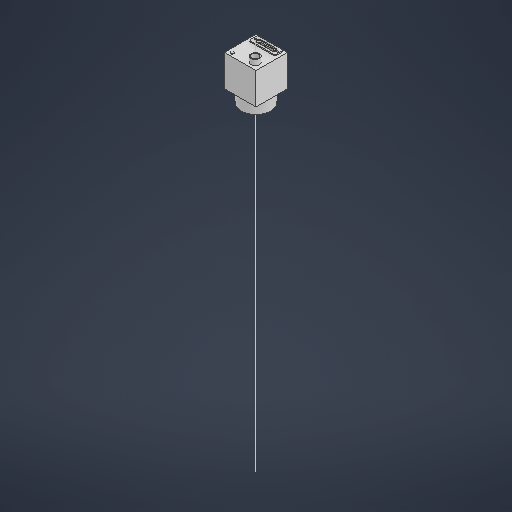
# Autodesk Inventor part: OpticalCamera
Saved by Autodesk Inventor 2026.2 (Build 302298000, 298)
## iProperties
Created: 2026-02-27
Part Number: OpticalCamera
Material: Generic
Document SubType Name: Modeling
Designer: mumin
Density: 1 g/cm^3
Appearance: Default
Author: mumin
Autodesk Inventor part; units mm, degrees
ref_plane "YZ Plane" through (0, 0, 0) normal (1, 0, 0) x (0, 1, 0)
ref_plane "XZ Plane" through (0, 0, 0) normal (0, 1, 0) x (-1, 0, 0)
sketch "Sketch1" plane through (0, 0, 0) normal (0, 1, 0) x (-1, 0, 0)
  line L0 (-15, -15) -> (15, -15)
  line L1 (15, -15) -> (15, 15)
  line L2 (15, 15) -> (-15, 15)
  line L3 (-15, 15) -> (-15, -15)
  line L4 (-15, -15) -> (15, 15) construction
  line L5 (15, -15) -> (-15, 15) construction
  point P0 (0, 0)
  dimension "d0" = 30
  dimension "d1" = 30
  constraints: 12 end point, 2 midpoint, 2 parallel, 1 horizontal, 1 perpendicular
  measures "d0" distance of L2.end L1.end
  measures "d1" distance of L1.end L0.end
extrude "Cube" add sketch "Sketch1" along normal blind 30
sketch "Sketch2" plane through (0, 0, 0) normal (0, -1, 0) x (1, 0, 0)
  circle A0 centre (0, 0) radius 14
  circle A1 centre (0, 0) radius 12.5
  dimension "d4" = 28
  dimension "d7" = 1.5
  constraints: 2 centre point, 1 coincident
  measures "d4" diameter of A0
  measures "d7" radial gap between concentric circles of A0 A1
extrude "Lens Mount" add sketch "Sketch2" along normal blind 11.3
sketch "Sketch3" plane through (0, 0, 0) normal (0, -1, 0) x (1, 0, 0)
  line L0 (7.5, -5) -> (-7.5, -5)
  line L1 (-7.5, -5) -> (-7.5, 5)
  line L2 (-7.5, 5) -> (7.5, 5)
  line L3 (7.5, 5) -> (7.5, -5)
  line L4 (7.5, -5) -> (-7.5, 5) construction
  line L5 (-7.5, -5) -> (7.5, 5) construction
  point P0 (0, 0)
  dimension "d8" = 15
  dimension "d9" = 10
  constraints: 12 end point, 2 midpoint, 2 parallel, 1 horizontal, 1 perpendicular
  measures "d8" distance of L1.end L2.end
  measures "d9" distance of L0.end L1.end
extrude "\"Sensor\"" cut sketch "Sketch3" against normal blind 2
sketch "Sketch4" plane through (15, 0, -15) normal (0, 0, -1) x (-1, 0, 0)
  line L0 (15, 0) -> (15, 30.669)
  line L1 (0, 30) -> (30, 30) projected
  point P0 (15, 26.85)
  point P1 (5, 3.15)
  point P2 (25, 3.15)
  dimension "d12" = 23.7
  dimension "d13" = 20
  dimension "d14" = 3.15
  constraints: 2 end point, 1 point on line, 1 symmetric about line
  measures "d12" vertical distance of point (15, 26.85) point (5, 3.15)
  measures "d13" distance of point (25, 3.15) point (5, 3.15)
  measures "d14" distance from line of L1 point (15, 26.85)
hole "Mounting Holes" at (0, 26.85, -15) at (10, 3.15, -15) at (-10, 3.15, -15) direction (0, 0, 1) diameter 3 depth 3 tip angle 118
sketch "Sketch5" plane through (0, 30, 0) normal (0, 1, 0) x (1, 0, 0)
  circle A0 centre (7.7053, -8.4968) radius 4
  circle A1 centre (7.7053, -8.4968) radius 3.2659
  point P0 (0, 0)
  dimension "d22" = 8
  constraints: 2 centre point
  measures "d22" diameter of A0
extrude "Cable Port" add sketch "Sketch5" along normal blind 5
sketch "Sketch6" plane through (0, 30, 0) normal (0, 1, 0) x (1, 0, 0)
  line L0 (7.2728, 8.793) -> (-7.0273, 8.793)
  line L1 (-7.0273, 8.793) -> (-6.3141, 10.6463)
  line L2 (-6.3141, 10.6463) -> (-2.7583, 10.6463)
  line L3 (-2.7583, 10.6463) -> (-2.3847, 9.4043)
  line L4 (-2.3847, 9.4043) -> (-1.5951, 9.4043)
  line L5 (-1.5951, 9.4043) -> (-1.2927, 10.6463)
  line L6 (-1.2927, 10.6463) -> (6.6007, 10.6463)
  line L7 (6.6007, 10.6463) -> (7.2728, 8.793)
  point P0 (0, 0)
  constraints: 16 end point, 2 parallel, 2 point on line, 1 horizontal
extrude "HDMI profile" cut sketch "Sketch6" against normal blind 3
sketch "Sketch8" plane through (0, 30, 0) normal (0, 1, 0) x (1, 0, 0)
  line L0 (-7.5, 11.8014) -> (7.5, 11.8014)
  line L1 (9, 10.3014) -> (9, 9.362)
  line L2 (7.5, 7.862) -> (-7.5, 7.862)
  line L3 (-9, 9.362) -> (-9, 10.3014)
  line L4 (-9, 11.8014) -> (9, 7.862) construction
  line L5 (9, 11.8014) -> (-9, 7.862) construction
  arc A0 (7.5, 7.862) -> (9, 9.362) centre (7.5, 9.362) ccw
  arc A1 (-9, 9.362) -> (-7.5, 7.862) centre (-7.5, 9.362) ccw
  arc A2 (-7.5, 11.8014) -> (-9, 10.3014) centre (-7.5, 10.3014) ccw
  arc A3 (9, 10.3014) -> (7.5, 11.8014) centre (7.5, 10.3014) ccw
  line L6 (-11.209, 13.8051) -> (11.209, 13.8051)
  line L7 (12.209, 12.8051) -> (12.209, 6.8583)
  line L8 (11.209, 5.8583) -> (-11.209, 5.8583)
  line L9 (-12.209, 6.8583) -> (-12.209, 12.8051)
  line L10 (-12.209, 13.8051) -> (12.209, 5.8583) construction
  line L11 (12.209, 13.8051) -> (-12.209, 5.8583) construction
  arc A4 (11.209, 5.8583) -> (12.209, 6.8583) centre (11.209, 6.8583) ccw
  arc A5 (-12.209, 6.8583) -> (-11.209, 5.8583) centre (-11.209, 6.8583) ccw
  arc A6 (-11.209, 13.8051) -> (-12.209, 12.8051) centre (-11.209, 12.8051) ccw
  arc A7 (12.209, 12.8051) -> (11.209, 13.8051) centre (11.209, 12.8051) ccw
  circle A8 centre (10.5, 9.8317) radius 0.75
  circle A9 centre (-10.5, 9.8317) radius 0.75
  point P0 (0, 0)
  point P1 (0, 9.8317)
  dimension "d27" = 1.5
  dimension "d28" = 1
  dimension "d31" = 24.4179
  dimension "d32" = 18
  dimension "d33" = 1.5
  dimension "d34" = 10.5
  dimension "d35" = 1.5
  dimension "d36" = 10.5
  constraints: 24 end point, 16 point on circle, 16 point on line, 16 tangent, 10 centre point, 6 equal radius, 4 midpoint, 4 parallel, 2 horizontal, 2 perpendicular
  measures "d27" radius of A0
  measures "d28" radius of A4
  measures "d31" distance between parallel lines of L9 L7
  measures "d32" distance between parallel lines of L1 L3
  measures "d33" diameter of A8
  measures "d34" distance of point (0, 9.832) A8.centre
  measures "d35" diameter of A9
  measures "d36" distance of point (0, 9.832) A9.centre
extrude "Cable Mount" add sketch "Sketch8" along normal blind 1
sketch "Sketch9" plane through (0, 30, 0) normal (0, 1, 0) x (1, 0, 0)
  circle A0 centre (-11.0721, -11.5458) radius 1.5
  point P0 (0, 0)
  dimension "d37" = 3
  constraints: 1 centre point
  measures "d37" diameter of A0
extrude "Extrusion7" cut sketch "Sketch9" against normal blind 0.5
ref_plane "Work Plane1" through (-11.0721, 29.5, 11.5458) normal (0, 0, 1) x (0, -1, 0)
sketch "Sketch10" plane through (-11.0721, 29.5, 11.5458) normal (0, 0, 1) x (0, -1, 0)
  line L0 (0, -1.5) -> (0, 1.5) projected
  line L1 (0, -1.5) -> (0, 1.5) projected
  line L2 (-0.5, -1.5) -> (-0.5, 1.5) projected
  line L3 (0, -1.5) -> (0, 1.5) projected
  line L4 (-1.5, 0) -> (0, 0)
  arc A0 (-1.5, 0) -> (0, -1.5) centre (0, 0) ccw
  line L5 (-14.76, 0) -> (50.06, 0) projected
  point P0 (29.5, 11.0721)
  point P1 (0, 0)
  constraints: 4 end point, 2 point on circle, 1 centre point, 1 horizontal, 1 midpoint
revolve "Revolution1" add sketch "Sketch10" angle 360 about axis through (-11.0721, 29.5, 11.5458) along (0, -1, 0)
body "Solid1"
